centerHolderBottom_v11 (Autodesk Fusion 360 design; units mm, degrees)
Autodesk Fusion 360 part; units mm, degrees
note: some values were not read from the file. Set by a fixed rule: which face or edge a step refers to.
sketch "Sketch1" plane through (0, 0, 0) normal (0, 0, 1) x (1, 0, 0)
  circle A0 centre (0, 0) radius 6.35
  dimension "d1" = 12.7
  constraint coincident A0.centre origin
  measures "d1" diameter of A0
extrude "Extrude1" add sketch "Sketch1" along normal blind 25.4
ref_plane "WorkPlane1" through (0, -6.35, 16.0163) normal (0, -1, 0) x (-1, 0, 0)
sketch "Sketch2" plane through (0, -6.35, 16.0163) normal (0, -1, 0) x (1, 0, 0)
  line L0 (6.35, 9.3837) -> (-6.35, 9.3837)
  line L1 (6.35, -16.0163) -> (-6.35, -16.0163)
  point P0 (0, 9.3837)
  constraint midpoint L0 P0
ref_plane "WorkPlane2" through (0, 0, 22.225) normal (0, 0, 1) x (1, 0, 0)
sketch "Sketch4" plane through (0, 0, 22.225) normal (0, 0, 1) x (1, 0, 0)
  circle A0 centre (0, 0) radius 6.35
  line L0 (0, 0) -> (0, -6.35) construction
  line L1 (0, 0) -> (5.4993, 3.175) construction
  line L2 (0, 0) -> (-5.4993, 3.175) construction
  dimension "d22" = 360
  constraint coincident A0.centre L0.start
  constraint coincident A0 L0.end
  constraint vertical L0
hole "Hole1" at (0, -6.35, 25.4) direction (0, 1, 0) diameter 6.35 depth 6.35 tip angle 180
pattern_circular "C-Pattern1" count 3 over 360 about axis through (0, 0, 0) along (0, 0, 1) of "Hole1"
extrude "Extrude2" cut sketch "Sketch4" against normal blind 0.127 from surface at 3.175
hole "Hole2" at (0, 0, 0) direction (0, 0, 1) diameter 2.2708 end up to surface (25.273 mm away)
thread "Thread1" "ANSI Unified Screw Threads 0.112(#4) 4-40 UNC 2B" major diameter 2.8448 minor diameter 2.2708 pitch 0.635 angle 60 resizes the face on face at (0.0837, 1.1323, 7.4558)
hole "Hole3" at (0, 0, 0) direction (0, 0, 1) diameter 5.1181 depth 19.05 tip angle 180
thread "Thread2" "ANSI Unified Screw Threads 0.25 1/4-20 UNC 1B"
equation "d5 = d1 / 2"
